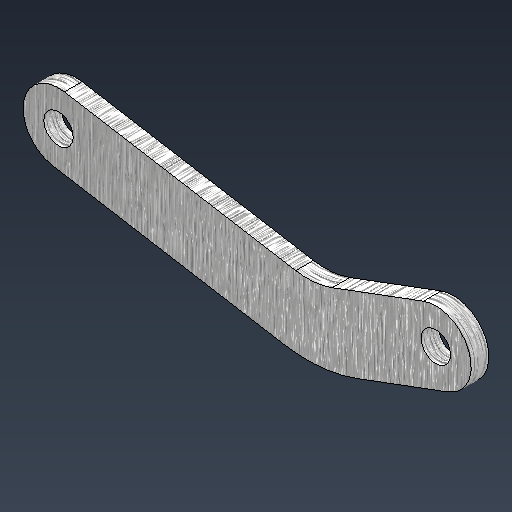
# Autodesk Inventor part: PLATE,LINK,FRONT,INTAKE
Saved by Autodesk Inventor 2026 (Build 300175050, 175E)
## iProperties
Created: 2026-02-15
Part Number: PLATE,LINK,FRONT,INTAKE
Material: Aluminum 7075
Document SubType Name: Modeling
Designer: Jthib
Mass: 232.773 g
Surface Area: 234.602 cm^2
Volume: 82.8375 cm^3
Density: 2.81 g/cm^3
Appearance: Satin - Brushed Heavy
Author: Jthib
Autodesk Inventor part; units mm, degrees
ref_plane "YZ Plane" through (0, 0, 0) normal (1, 0, 0) x (0, 1, 0)
ref_plane "XZ Plane" through (0, 0, 0) normal (0, 1, 0) x (-1, 0, 0)
ref_plane "XY Plane" through (0, 0, 0) normal (0, 0, 1) x (1, 0, 0)
sketch "Sketch1" plane through (0, 0, 0) normal (0, 0, 1) x (1, 0, 0)
  line L0 (-101.6, 0) -> (101.6, 0) construction
  arc A0 (-98.4242, 18.7834) -> (-104.7758, -18.7834) centre (-101.6, 0) ccw
  arc A1 (108.2414, -17.8548) -> (94.9586, 17.8548) centre (101.6, 0) ccw
  line L1 (108.2414, -17.8548) -> (59.0939, -36.136)
  line L2 (19.8252, -39.8504) -> (-104.7758, -18.7834)
  line L3 (-98.4242, 18.7834) -> (26.1768, -2.2835)
  line L4 (45.8112, -0.4263) -> (94.9586, 17.8548)
  line L5 (36.2428, -3.9854) -> (39.9572, -43.2542) construction
  line L6 (38.1, -23.6198) -> (-101.6, 0) construction
  line L7 (38.1, -23.6198) -> (101.6, 0) construction
  arc A2 (19.8252, -39.8504) -> (59.0939, -36.136) centre (32.5284, 35.2833) ccw
  arc A3 (26.1768, -2.2835) -> (45.8112, -0.4263) centre (32.5284, 35.2833) ccw
  point P0 (0, 0)
  dimension "d1" = 38.1
  dimension "d2" = 203.2
  dimension "d12" = 150
  dimension "d13" = 63.5
  dimension "d14" = 76.2
  constraints: 18 end point, 8 point on circle, 8 tangent, 4 centre point, 4 point on line, 2 midpoint, 2 parallel, 1 concentric, 1 equal radius, 1 horizontal
  measures "d1" diameter of A0
  measures "d2" distance of L0.start L0.end
  measures "d12" angle of L7 L6
  measures "d13" horizontal distance of L6.start L0.end
  measures "d14" radius of A2
extrude "Extrusion1" add sketch "Sketch1" along normal mid plane 9.525
sketch "Sketch2" plane through (0, 0, 4.7625) normal (0, 0, 1) x (1, 0, 0)
  arc A0 (-98.4242, 18.7834) -> (-104.7758, -18.7834) centre (-101.6, 0) ccw construction
  arc A1 (108.2414, -17.8548) -> (94.9586, 17.8548) centre (101.6, 0) ccw construction
  point P0 (0, 0)
  constraints: 2 coincident
hole "Hole1" at (-101.6, 0, 4.7625) at (101.6, 0, 4.7625) direction (0, 0, -1) diameter 15.875 end through all start extended yes
body "Solid1"
